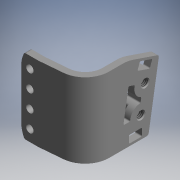
# Autodesk Inventor part: 3899099 DHAS-MA-B6-80---(winkel)
Saved by Autodesk Inventor 2017.3 (Build 213256000, 256)
## iProperties
Part Number: 3899099 DHAS-MA-B6-80---(winkel)
Material: Generic
Catalog Web Link: www.cadenas.de
Description: DHAS-MA_w-bracket
Vendor: FESTO
Document SubType Name: Modeling
Designer: partserver
Manufacturer: FESTO
Mass: 5.29381 g
Surface Area: 44.3897 cm^2
Volume: 5.29381 cm^3
Density: 1 g/cm^3
Appearance: PSOLRGB-175-175-175
Category: PARTsolutions
Company: FESTO
Title: 3899099 DHAS-MA-B6-80---(winkel)
Author: Cadenas PARTsolutions
Comments: bracket
PSOL_IDENT_0: {$CADENAS_DATA\23d-libs\festo\parts\d\dhas\parts\dhas_ma_winkel.prj},208 {VTYP=3D},{NB=3899099 DHAS-
PSOL_IDENT_1: MA-B6-80---(winkel)},{LINA=3899099 DHAS-MA-B6-80---(winkel)},{NN=DHAS-MA_w},{DATE=30.08.2019 14:48:2
PSOL_IDENT_2: 6},{GEOMDATE=01.09.2017 11:45:00},{VERSION=},{LINEID=230},{WBVAR=},{WBNUMERIC=}  {NB=3899099 DHAS-MA
PSOL_IDENT_3: -B6-80---(winkel)},{LINA=3899099 DHAS-MA-B6-80---(winkel)},{KT=DUMMY},{TNR=3899099},{TYP=DHAS-MA-B6-
PSOL_IDENT_4: 80},{SIZE=80}
NB: 3899099 DHAS-MA-B6-80---(winkel)
NN: DHAS-MA_w
NT: bracket
NBSYN: $TNR. $TYP.---(winkel)
LINA: 3899099 DHAS-MA-B6-80---(winkel)
CATALOG: Festo
TNR: 3899099
TYP: DHAS-MA-B6-80
SIZE: 80
SUPPLIER: FESTO
ARTICLENO: 3899099 DHAS-MA-B6-80---(winkel)
BOMINFO: 3899099 DHAS-MA-B6-80---(winkel)
CREATOR: CADENAS GmbH
Autodesk Inventor part; units mm, degrees
ref_plane "YZ Plane" through (0, 0, 0) normal (1, 0, 0) x (0, 1, 0)
ref_plane "XZ Plane" through (0, 0, 0) normal (0, 1, 0) x (-1, 0, 0)
ref_plane "XY Plane" through (0, 0, 0) normal (0, 0, 1) x (1, 0, 0)
sketch "Sketch_3" plane through (0, 0, 0) normal (0, 0, 1) x (1, 0, 0)
  line L0 (0, 1.811) -> (20.7, 0)
  line L1 (20.7, 0) -> (28.6, 0)
  line L2 (28.6, 0) -> (28.6, 3)
  line L3 (28.6, 3) -> (20.7, 3)
  line L4 (20.7, 3) -> (3, 4.5485)
  line L5 (3, 4.5485) -> (3, 35)
  line L6 (3, 35) -> (0, 35)
  line L7 (0, 35) -> (0, 1.811)
  constraints: 16 end point
extrude "Extrusion1" add sketch "Sketch_3" along normal blind 34.5
sketch "Sketch_2" plane through (0, 0, 0) normal (0, 0, 1) x (1, 0, 0)
  line L0 (0, 1.811) -> (20.7, 0)
  line L1 (20.7, 0) -> (28.6, 0)
  line L2 (28.6, 0) -> (28.6, 3)
  line L3 (28.6, 3) -> (21.0493, 3)
  arc A0 (20.352, 3.0304) -> (21.0493, 3) centre (21.0493, 11) ccw
  line L4 (20.352, 3.0304) -> (10.3028, 3.9096)
  arc A1 (3, 11.8792) -> (10.3028, 3.9096) centre (11, 11.8792) ccw
  line L5 (3, 11.8792) -> (3, 35)
  line L6 (3, 35) -> (0, 35)
  line L7 (0, 35) -> (0, 1.811)
  constraints: 16 end point, 4 point on circle, 2 centre point
extrude "Extrusion2" add sketch "Sketch_2" along normal blind 34.5
sketch "Sketch_4" plane through (0, 0, 0) normal (0, 0, 1) x (1, 0, 0)
  line L0 (-5, -5) -> (35, -5)
  line L1 (35, -5) -> (35, 45)
  line L2 (35, 45) -> (-5, 45)
  line L3 (-5, 45) -> (-5, -5)
  arc A0 (0, 11.8907) -> (10.0413, 0.9325) centre (11, 11.8907) ccw
  line L4 (10.0413, 0.9325) -> (20.2216, 0.0419)
  arc A1 (20.2216, 0.0419) -> (21.1803, 0) centre (21.1803, 11) ccw
  line L5 (21.1803, 0) -> (28.6, 0)
  line L6 (28.6, 0) -> (28.6, 3)
  line L7 (28.6, 3) -> (21.0493, 3)
  arc A2 (20.352, 3.0304) -> (21.0493, 3) centre (21.0493, 11) ccw
  line L8 (20.352, 3.0304) -> (10.3028, 3.9096)
  arc A3 (3, 11.8792) -> (10.3028, 3.9096) centre (11, 11.8792) ccw
  line L9 (3, 11.8792) -> (3, 35)
  line L10 (3, 35) -> (0, 35)
  line L11 (0, 35) -> (0, 11.8907)
  constraints: 24 end point, 8 point on circle, 4 centre point
extrude "Extrusion3" cut sketch "Sketch_4" along normal blind 48
sketch "Sketch_5" plane through (0, 0, 0) normal (1, 0, 0) x (0, 1, 0)
  line L0 (45, 55) -> (-5, 55)
  line L1 (-5, 55) -> (-5, -5)
  line L2 (-5, -5) -> (45, -5)
  line L3 (45, -5) -> (45, 55)
  line L4 (29.2518, 34.5) -> (0, 34.5)
  line L5 (0, 34.5) -> (0, 0)
  line L6 (0, 0) -> (18.1302, 0)
  arc A0 (18.1302, 0) -> (22.9394, 0.7918) centre (18.1302, 15) ccw
  line L7 (22.9394, 0.7918) -> (34.1954, 4.6018)
  arc A1 (34.1954, 4.6018) -> (34.8614, 5.7122) centre (33.8748, 5.549) ccw
  line L8 (34.8614, 5.7122) -> (30.2384, 33.6632)
  arc A2 (30.2384, 33.6632) -> (29.2518, 34.5) centre (29.2518, 33.5) ccw
  constraints: 18 end point, 6 point on circle, 3 centre point
extrude "Extrusion4" cut sketch "Sketch_5" along normal blind 3
sketch "Sketch_6" plane through (0, 0, 0) normal (0, 1, 0) x (-1, 0, 0)
  line L0 (5, 53) -> (-35, 53)
  line L1 (-35, 53) -> (-35, -5)
  line L2 (-35, -5) -> (5, -5)
  line L3 (5, -5) -> (5, 53)
  line L4 (0, 34.5) -> (-26.4831, 34.5)
  arc A0 (-26.4831, 34.5) -> (-27.388, 33.9255) centre (-26.4831, 33.5) ccw
  arc A1 (-27.388, 33.9255) -> (-28.6, 28.5) centre (-15.85, 28.5) ccw
  line L5 (-28.6, 28.5) -> (-28.6, 6)
  arc A2 (-28.6, 6) -> (-27.388, 0.5745) centre (-15.85, 6) ccw
  arc A3 (-27.388, 0.5745) -> (-26.4831, 0) centre (-26.4831, 1) ccw
  line L6 (-26.4831, 0) -> (0, 0)
  line L7 (0, 0) -> (0, 34.5)
  constraints: 16 end point, 8 point on circle, 4 centre point
extrude "Extrusion5" cut sketch "Sketch_6" along normal blind 3
sketch "Sketch6" plane through (21.1803, 0, 0) normal (0, -1, 0) x (1, 0, 0)
  point P0 (3.4197, 29.25)
hole "Hole1" at (24.6, 0, 29.25) direction (0, 1, 0) diameter 3.4 depth 3
pattern_linear "Rectangular Pattern1" count 4 spacing 8 along (0, 0, -1) of "Hole1"
sketch "Sketch_10" plane through (0, 0, 0) normal (1, 0, 0) x (0, 1, 0)
  arc A0 (30.8781, 7.7408) -> (30.2437, 8.0531) centre (30.4047, 7.5797) ccw
  line L0 (30.2437, 8.0531) -> (25.5102, 6.4425)
  arc A1 (25.5102, 6.4425) -> (25.1979, 5.808) centre (25.6712, 5.9691) ccw
  line L1 (25.1979, 5.808) -> (26.0032, 3.4413)
  arc A2 (26.0032, 3.4413) -> (26.6376, 3.129) centre (26.4765, 3.6024) ccw
  line L2 (26.6376, 3.129) -> (31.3711, 4.7396)
  arc A3 (31.3711, 4.7396) -> (31.6834, 5.374) centre (31.21, 5.213) ccw
  line L3 (31.6834, 5.374) -> (30.8781, 7.7408)
  constraints: 8 end point, 8 point on circle, 4 centre point
extrude "Extrusion6" cut sketch "Sketch_10" along normal blind 3
sketch "Sketch_18" plane through (0, 0, 0) normal (1, 0, 0) x (0, 1, 0)
  arc A0 (21.621, 33.4596) -> (21.121, 32.9597) centre (21.621, 32.9596) ccw
  line L0 (21.121, 32.9597) -> (21.1206, 30.4597)
  arc A1 (21.1206, 30.4597) -> (21.6205, 29.9596) centre (21.6206, 30.4596) ccw
  line L1 (21.6205, 29.9596) -> (26.6205, 29.9589)
  arc A2 (26.6205, 29.9589) -> (27.1206, 30.4588) centre (26.6206, 30.4589) ccw
  line L2 (27.1206, 30.4588) -> (27.121, 32.9588)
  arc A3 (27.121, 32.9588) -> (26.621, 33.4589) centre (26.621, 32.9589) ccw
  line L3 (26.621, 33.4589) -> (21.621, 33.4596)
  constraints: 8 end point, 8 point on circle, 4 centre point
extrude "Extrusion7" cut sketch "Sketch_18" along normal blind 3
sketch "Sketch_12" plane through (0, 0, 0) normal (1, 0, 0) x (0, 1, 0)
  line L0 (21.1607, 24.7868) -> (19.1193, 24.7853)
  arc A0 (19.1193, 24.7853) -> (18.6264, 24.2037) centre (19.1196, 24.2853) ccw
  line L1 (18.6264, 24.2037) -> (20.8221, 10.9278)
  arc A1 (20.8221, 10.9278) -> (21.4761, 10.5359) centre (21.3154, 11.0093) ccw
  line L2 (21.4761, 10.5359) -> (23.4093, 11.1918)
  arc A2 (23.4093, 11.1918) -> (23.7348, 11.7822) centre (23.2486, 11.6653) ccw
  arc A3 (26.4658, 17.4751) -> (23.7348, 11.7822) centre (28.5961, 12.9516) ccw
  arc A4 (26.4658, 17.4751) -> (26.746, 18.009) centre (26.2527, 17.9274) ccw
  line L3 (26.746, 18.009) -> (26.5148, 19.407)
  arc A5 (26.5148, 19.407) -> (26.0776, 19.8223) centre (26.0215, 19.3254) ccw
  arc A6 (21.659, 24.3326) -> (26.0776, 19.8223) centre (26.6379, 24.7907) ccw
  arc A7 (21.659, 24.3326) -> (21.1607, 24.7868) centre (21.1611, 24.2868) ccw
  constraints: 16 point on circle, 8 centre point, 8 end point
extrude "Extrusion8" cut sketch "Sketch_12" along normal blind 3
sketch "Sketch_20" plane through (3, 0, 0) normal (1, 0, 0) x (0, 0, -1)
  arc A0 (-28.9551, 23.5808) -> (-27.7919, 22.594) centre (-27.9551, 23.5806) ccw
  line L0 (-27.7919, 22.594) -> (-21.139, 23.6944)
  arc A1 (-21.139, 23.6944) -> (-20.43, 24.1917) centre (-21.3022, 24.681) ccw
  arc A2 (-20.43, 24.1917) -> (-19.8223, 26.0776) centre (-24.7907, 26.6379) ccw
  arc A3 (-19.407, 26.5148) -> (-19.8223, 26.0776) centre (-19.3254, 26.0215) ccw
  line L1 (-19.407, 26.5148) -> (-18.009, 26.746)
  arc A4 (-17.4751, 26.4658) -> (-18.009, 26.746) centre (-17.9274, 26.2527) ccw
  arc A5 (-17.4751, 26.4658) -> (-16.2925, 24.8761) centre (-12.9516, 28.5961) ccw
  arc A6 (-16.2925, 24.8761) -> (-15.4611, 24.6335) centre (-15.6243, 25.6201) ccw
  line L2 (-15.4611, 24.6335) -> (-8.8082, 25.7339)
  arc A7 (-8.8082, 25.7339) -> (-8.0246, 27.0426) centre (-8.9713, 26.7204) ccw
  line L3 (-8.0246, 27.0426) -> (-9.6572, 31.8405)
  arc A8 (-9.6572, 31.8405) -> (-10.7671, 32.505) centre (-10.6039, 31.5184) ccw
  line L4 (-10.7671, 32.505) -> (-18.316, 31.2564)
  arc A9 (-18.316, 31.2564) -> (-18.641, 30.9492) centre (-18.2507, 30.8618) ccw
  arc A10 (-18.9661, 30.6421) -> (-18.641, 30.9492) centre (-19.0313, 31.0367) ccw
  line L5 (-18.9661, 30.6421) -> (-19.7553, 30.5115)
  arc A11 (-20.162, 30.6977) -> (-19.7553, 30.5115) centre (-19.8206, 30.9062) ccw
  arc A12 (-20.162, 30.6977) -> (-20.5686, 30.8838) centre (-20.5033, 30.4892) ccw
  line L6 (-20.5686, 30.8838) -> (-28.1175, 29.6353)
  arc A13 (-28.1175, 29.6353) -> (-28.9544, 28.6488) centre (-27.9544, 28.6487) ccw
  line L7 (-28.9544, 28.6488) -> (-28.9551, 23.5808)
  constraints: 28 point on circle, 16 end point, 14 centre point
extrude "Extrusion9" add sketch "Sketch_20" along normal blind 3
sketch "Sketch_13" plane through (0, 25.167, 33.6841) normal (0, -0.9865978, -0.163171) x (1, 0, 0)
  line L0 (6, -9.014) -> (0, -9.014)
  line L1 (0, -9.014) -> (0, -7.014)
  line L2 (0, -7.014) -> (0.379, -7.393)
  line L3 (0.379, -7.393) -> (5.621, -7.393)
  line L4 (5.621, -7.393) -> (6, -7.014)
  line L5 (6, -7.014) -> (6, -9.014)
  line L6 (6, -9.014) -> (0, -9.014)
  constraints: 14 end point
revolve "Revolution1" cut sketch "Sketch_13" angle 360 about axis through (6, 26.6378, 24.791) along (1, 0, 0)
thread "Thread1" size "M4x0.7" class "6H" standard "ISO Metric profile" full length
sketch "Sketch_14" plane through (0, 25.167, 33.6841) normal (0, -0.9865978, -0.163171) x (1, 0, 0)
  line L0 (6, -21.014) -> (0, -21.014)
  line L1 (0, -21.014) -> (0, -19.014)
  line L2 (0, -19.014) -> (0.379, -19.393)
  line L3 (0.379, -19.393) -> (5.621, -19.393)
  line L4 (5.621, -19.393) -> (6, -19.014)
  line L5 (6, -19.014) -> (6, -21.014)
  line L6 (6, -21.014) -> (0, -21.014)
  constraints: 14 end point
revolve "Revolution2" cut sketch "Sketch_14" angle 360 about axis through (6, 28.5959, 12.9518) along (1, 0, 0)
thread "Thread2" size "M4x0.7" class "6H" standard "ISO Metric profile" full length
ref_plane "ANBAU_XY" through (0, 0, 0) normal (0, 0, 1) x (1, 0, 0)
ref_plane "ANBAU_YZ" through (0, 0, 0) normal (1, 0, 0) x (0, 1, 0)
ref_plane "ANBAU_ZX" through (0, 0, 0) normal (0, 1, 0) x (0, 0, 1)
ref_plane "DIN912_1_XY" through (24.6, 3, 29.25) normal (0, 1, 0) x (1, 0, 0)
ref_plane "DIN912_1_YZ" through (24.6, 3, 29.25) normal (1, 0, 0) x (0, 0, -1)
ref_plane "DIN912_1_ZX" through (24.6, 3, 29.25) normal (0, 0, -1) x (0, 1, 0)
ref_plane "DIN912_2_XY" through (24.6, 3, 21.25) normal (0, 1, 0) x (1, 0, 0)
ref_plane "DIN912_2_YZ" through (24.6, 3, 21.25) normal (1, 0, 0) x (0, 0, -1)
ref_plane "DIN912_2_ZX" through (24.6, 3, 21.25) normal (0, 0, -1) x (0, 1, 0)
ref_plane "DIN912_3_XY" through (24.6, 3, 13.25) normal (0, 1, 0) x (1, 0, 0)
ref_plane "DIN912_3_YZ" through (24.6, 3, 13.25) normal (1, 0, 0) x (0, 0, -1)
ref_plane "DIN912_3_ZX" through (24.6, 3, 13.25) normal (0, 0, -1) x (0, 1, 0)
body "Solid1"
